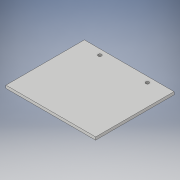
# Autodesk Inventor part: mainboard
Saved by Autodesk Inventor 2018 (Build 220112000, 112)
## iProperties
Created: 2017-12-03
Part Number: mainboard
Material: Generic
Document SubType Name: Modeling
Designer: Cole Tucker
Density: 1 g/cm^3
Appearance: Default
Author: Cole Tucker
Autodesk Inventor part; units mm, degrees
ref_plane "YZ Plane" through (0, 0, 0) normal (1, 0, 0) x (0, 1, 0)
ref_plane "XZ Plane" through (0, 0, 0) normal (0, 1, 0) x (-1, 0, 0)
ref_plane "XY Plane" through (0, 0, 0) normal (0, 0, 1) x (1, 0, 0)
sketch "Sketch1" plane through (0, 0, 0) normal (0, 1, 0) x (-1, 0, 0)
  line L0 (0, 0) -> (-101.6, 0)
  line L1 (-101.6, 0) -> (-101.6, -88.9)
  line L2 (-101.6, -88.9) -> (0, -88.9)
  line L3 (0, -88.9) -> (0, 0)
  line L4 (-50.8, -88.9) -> (-23.8125, -88.9)
  line L5 (-50.8, -88.9) -> (-77.7875, -88.9)
  line L6 (-77.7875, -88.9) -> (-77.7875, -82.55)
  line L7 (-23.8125, -88.9) -> (-23.8125, -82.55)
  circle A0 centre (-23.8125, -82.55) radius 1.905
  circle A1 centre (-77.7875, -82.55) radius 1.905
  dimension "d0" = 101.6
  dimension "d1" = 88.9
  dimension "d2" = 26.9875
  dimension "d3" = 26.9875
  dimension "d4" = 6.35
  dimension "d5" = 6.35
  dimension "d6" = 3.81
  dimension "d7" = 3.81
  constraints: 16 end point, 2 centre point, 2 coincident, 2 parallel, 2 perpendicular, 2 point on line, 1 horizontal, 1 midpoint, 1 vertical
  measures "d0" distance of L2.end L1.end
  measures "d1" distance of L1.end L0.end
  measures "d2" distance of L4.start L4.end
  measures "d3" distance of L4.start L5.end
  measures "d4" distance of L5.end L6.end
  measures "d5" distance of L4.end L7.end
  measures "d6" diameter of A0
  measures "d7" diameter of A1
extrude "Extrusion1" add sketch "Sketch1" along normal blind 3.175
body "Solid1"
